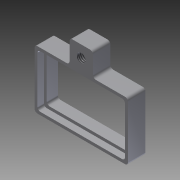
# Autodesk Inventor part: base
Saved by Autodesk Inventor 2011 (Build 150239000, 239)
## iProperties
Created: 2011-02-16
Part Number: base
Document SubType Name: Modeling
Designer: labuser
Density: 1 g/cm^3
Author: labuser
Autodesk Inventor part; units mm, degrees
ref_plane "YZ Plane" through (0, 0, 0) normal (1, 0, 0) x (0, 1, 0)
ref_plane "XZ Plane" through (0, 0, 0) normal (0, 1, 0) x (-1, 0, 0)
ref_plane "XY Plane" through (0, 0, 0) normal (0, 0, 1) x (1, 0, 0)
sketch "Sketch1" plane through (0, 0, 0) normal (0, 0, 1) x (1, 0, 0)
  line L0 (0, 0) -> (16, 0)
  line L1 (16, 0) -> (16, 10)
  line L2 (16, 10) -> (0, 10)
  line L3 (0, 10) -> (0, 0)
  dimension "d0" = 16
  dimension "d1" = 10
  constraints: 8 end point, 2 parallel, 1 horizontal, 1 perpendicular
  measures "d0" distance of L2.end L1.end
  measures "d1" distance of L1.end L0.end
extrude "Extrusion1" add sketch "Sketch1" along normal blind 3
sketch "Sketch2" plane through (0, 0, 3) normal (0, 0, 1) x (1, 0, 0)
  line L0 (1, 1) -> (15, 1)
  line L1 (15, 1) -> (15, 9)
  line L2 (15, 9) -> (1, 9)
  line L3 (1, 9) -> (1, 1)
  dimension "d4" = 14
  dimension "d5" = 8
  constraints: 8 end point, 2 parallel, 1 horizontal, 1 perpendicular
  measures "d4" distance of L2.end L1.end
  measures "d5" distance of L1.end L0.end
extrude "Extrusion2" cut sketch "Sketch2" against normal through all
sketch "Sketch3" plane through (0, 10, 0) normal (0, 1, 0) x (1, 0, 0)
  line L0 (0, -3) -> (16, -3) projected
  line L1 (16, 0) -> (0, 0) projected
  line L2 (0, 0) -> (0, -3) projected
  line L3 (6, -3) -> (10, -3)
  line L4 (10, -3) -> (10, 0)
  line L5 (10, 0) -> (6, 0)
  line L6 (6, 0) -> (6, -3)
  dimension "d13" = 4
  dimension "d14" = 6
  constraints: 8 end point, 2 parallel, 2 point on line, 1 horizontal, 1 perpendicular
  measures "d13" distance of L5.end L4.end
  measures "d14" distance between parallel lines of L6 L2
extrude "Extrusion3" add sketch "Sketch3" along normal blind 4 contours L6 L1 L4 L0
sketch "Sketch5" plane through (0, 0, 3) normal (0, 0, 1) x (1, 0, 0)
  line L0 (15, 9) -> (15, 1) projected
  line L1 (15, 1) -> (1, 1) projected
  line L2 (1, 1) -> (1, 9) projected
  line L3 (1, 9) -> (15, 9) projected
  line L4 (0.5, 9.5) -> (0.5, 0.5)
  line L5 (0.5, 0.5) -> (15.5, 0.5)
  line L6 (15.5, 0.5) -> (15.5, 9.5)
  line L7 (15.5, 9.5) -> (0.5, 9.5)
  dimension "d17" = 0.5
  constraints: 8 end point, 3 other
  measures "d17" distance between parallel lines of L4 L2
extrude "Extrusion4" cut sketch "Sketch5" against normal blind 1.1
sketch "Sketch6" plane through (0, 0, 3) normal (0, 0, 1) x (1, 0, 0)
  point P0 (8, 12)
hole "Hole1" at (8, 12, 3) direction (0, 0, -1) diameter 1.524 end through all
thread "Thread1" size "0-80 UNF" class "2B" standard "ANSI Unified Screw Threads" full length
sketch "Sketch7" plane through (0, 0, 0) normal (0, -1, 0) x (1, 0, 0)
  line L0 (0, 0) -> (0, 3) projected
  line L1 (0, 0) -> (16, 0) projected
  line L2 (7, 0) -> (9, 0)
  line L3 (9, 0) -> (9, 1)
  line L4 (9, 1) -> (7, 1)
  line L5 (7, 1) -> (7, 0)
  dimension "d29" = 2
  dimension "d30" = 1
  dimension "d31" = 7
  constraints: 8 end point, 2 parallel, 1 horizontal, 1 perpendicular, 1 point on line
  measures "d29" distance of L4.end L3.end
  measures "d30" distance of L3.end L2.end
  measures "d31" distance between parallel lines of L5 L0
extrude "Extrusion5" add sketch "Sketch7" along normal blind 1
fillet "Fillet1" radius 0.5 18 edges at (0.5, 0.5, 2.45) (1, 1, 0.95) (1, 9, 0.95) (0.5, 9.5, 2.45) (15, 9, 0.95) (15.5, 9.5, 2.45) (15, 1, 0.95) (15.5, 0.5, 2.45) (16, 0, 1.5) (9, 0, 0.5) (0, 0, 1.5) (7, 0, 0.5) (0, 10, 1.5) (6, 10, 1.5) (6, 14, 1.5) (10, 14, 1.5) (10, 10, 1.5) (16, 10, 1.5)
body "Solid1"
